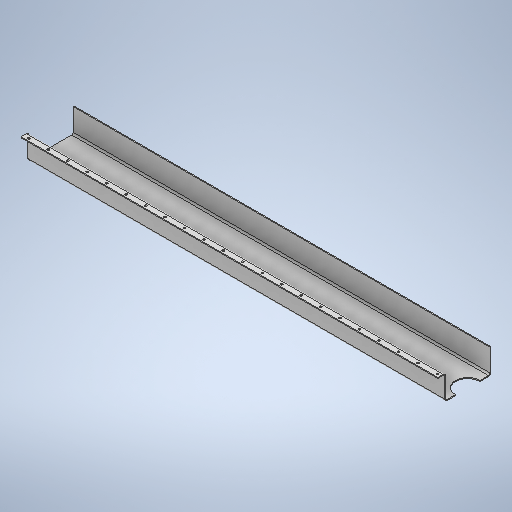
# Autodesk Inventor part: MSC 081 pillar 1
Saved by Autodesk Inventor 2025 (Build 290162010, 162A)
## iProperties
Created: 2024-06-25
Part Number: MSC 081 pillar 1
Material: Stainless Steel
Document SubType Name: Sheet Metal
Designer: admin
Density: 8 g/cm^3
Sheet Metal Rule: AISI304 3mm Die 32
Appearance: Default
Author: admin
Autodesk Inventor part; units mm, degrees
ref_plane "YZ Plane" through (0, 0, 0) normal (1, 0, 0) x (0, 1, 0)
ref_plane "XZ Plane" through (0, 0, 0) normal (0, 1, 0) x (-1, 0, 0)
ref_plane "XY Plane" through (0, 0, 0) normal (0, 0, 1) x (1, 0, 0)
sketch3d "3D Sketch1"
sketch "Sketch1" plane through (0, 0, 0) normal (0, 0, 1) x (1, 0, 0)
  line L0 (-675, 75) -> (675, 75)
  line L1 (675, 75) -> (675, -75)
  line L2 (675, -75) -> (-675, -75)
  line L3 (-675, -75) -> (-675, 75)
  line L4 (-675, 75) -> (675, -75) construction
  line L5 (675, 75) -> (-675, -75) construction
  point P0 (0, 0)
  dimension "d5" = 1350
  dimension "d30" = 150
  measures "d5" distance of L1.end L2.end
  measures "d30" distance of L2.end L0.start
extrude "Plate1" add sketch "Sketch1" along normal blind 3
sketch "Sketch6" plane through (675, -72, 0) normal (0, -1, 0) x (1, 0, 0)
  line L0 (-1350, 0) -> (0, 0)
  line L1 (0, 0) -> (0, 80)
  line L2 (0, 80) -> (-1350, 80)
  line L3 (-1350, 80) -> (-1350, 0)
  constraints: 6 end point, 1 horizontal, 1 perpendicular, 1 vertical
edge flange "Flange4" height 80 angle 90 thickness 3 bend radius 5 thickness toward (0, -1, 0) relief round relief width 3 relief depth 1.5 corner gap 5 corner form 0 edges at (0, -75, 3) (0, 75, 3) wall of the first edge with corners at (-675, -72, 0) (675, -72, 0) (675, -72, 80) (-675, -72, 80)
bend "Bend4"
corner "Corner4"
sketch "Sketch7" plane through (0, 0, 3) normal (0, 0, 1) x (1, 0, 0)
  circle A0 centre (675, 0) radius 40
  line L0 (675, 67) -> (675, -67) projected
  point P0 (0, 0)
  point P1 (675, -40)
  point P2 (675, 40)
  dimension "d70" = 80
  constraints: 1 centre point, 1 midpoint
  measures "d70" diameter of A0
extrude "Extrusion2" cut sketch "Sketch7" against normal through all contours L0 A0 picked at (666.8047, -12.472)
sketch "Sketch8" plane through (0, 0, 0) normal (0, 1, 0) x (-1, 0, 0)
  line L0 (675, 8) -> (-675, 8) construction
  line L1 (-675, 80) -> (-675, 8) construction
  line L2 (675, 80) -> (-675, 80) construction
  line L3 (675, 8) -> (675, 80) projected
  circle A0 centre (-655, 70) radius 2.5
  point P0 (0, 0)
  dimension "d73" = 5
  dimension "d74" = 10
  dimension "d75" = 20
  constraints: 1 centre point
  measures "d73" diameter of A0
  measures "d74" distance from line of L2 A0.centre
  measures "d75" distance from line of L1 A0.centre
extrude "Extrusion3" [suppressed]
pattern_linear "Rectangular Pattern1" [suppressed]
sketch "Sketch9" plane through (-675, -72, 77) normal (0, 0, 1) x (1, 0, 0)
  line L0 (1350, 0) -> (0, 0)
  line L1 (0, 0) -> (0, -25)
  line L2 (0, -25) -> (1350, -25)
  line L3 (1350, -25) -> (1350, 0)
  constraints: 6 end point, 1 horizontal, 1 perpendicular, 1 vertical
edge flange "Flange5" height 25 angle 90 thickness 3 bend radius 5 thickness toward (0, 0, 1) relief round relief width 3 relief depth 1.5 edges at (0, -75, 80) wall of the first edge with corners at (675, -72, 77) (-675, -72, 77) (-675, -97, 77) (675, -97, 77)
bend "Bend5"
corner "Corner5"
sketch "Sketch10" plane through (-675, -97, 80) normal (0, 0, 1) x (1, 0, 0)
  line L0 (1350, 17) -> (0, 17) projected
  line L1 (0, 0) -> (0, 17) projected
  line L2 (1350, 0) -> (0, 0) projected
  line L3 (1350, 17) -> (1350, 0) projected
  circle A0 centre (1340, 8.5) radius 3.5
  point P0 (675, 97)
  point P1 (1350, 8.5)
  dimension "d91" = 7
  dimension "d92" = 10
  constraints: 1 centre point, 1 horizontal alignment, 1 midpoint
  measures "d91" diameter of A0
  measures "d92" distance from line of L3 A0.centre
extrude "Cut1" cut sketch "Sketch10" against normal blind 3 contours A0
pattern_linear "Rectangular Pattern2" count 30 spacing 63 along (-1, 0, 0) of "Cut1"
equation "\"d93\" = Thickness"
equation "\"d6\" = Thickness"
equation "\"d60\" = BendReliefWidth"
equation "\"d61\" = BendReliefDepth"
equation "\"d62\" = MinimumRemnant"
equation "\"d63\" = TransitionRadius"
equation "\"d66\" = BendRadius"
equation "\"d67\" = CornerReliefSize"
equation "\"d68\" = GapSize"
equation "\"d69\" = JacobiRadiusSize"
equation "\"d81\" = BendReliefWidth"
equation "\"d82\" = BendReliefDepth"
equation "\"d83\" = MinimumRemnant"
equation "\"d84\" = TransitionRadius"
equation "\"d87\" = BendRadius"
equation "\"d88\" = CornerReliefSize"
equation "\"d89\" = GapSize"
equation "\"d90\" = JacobiRadiusSize"
equation "\"BendReliefWidth\" = Thickness"
equation "\"BendReliefDepth\" = 0.5 * Thickness"
equation "\"CornerReliefSize\" = 4 * Thickness"
equation "\"MinimumRemnant\" = 2 * Thickness"
equation "\"TransitionRadius\" = BendRadius"
equation "\"JacobiRadiusSize\" = BendRadius"
equation "\"GapSize\" = Thickness"
equation "\"Thickness\" = 3"
equation "\"BendRadius\" = 5"
body "Solid1"
